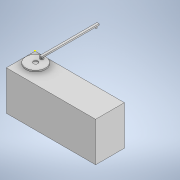
# Autodesk Inventor part: fnal
Saved by Autodesk Inventor 2021 (Build 250183000, 183)
## iProperties
Created: 2021-03-07
Part Number: fnal
Material: Generic
Document SubType Name: Modeling
Designer: V.Basavaraj
Density: 1 g/cm^3
Appearance: Default
Author: V.Basavaraj
Autodesk Inventor part; units mm, degrees
ref_plane "YZ Plane" through (0, 0, 0) normal (1, 0, 0) x (0, 1, 0)
ref_plane "XZ Plane" through (0, 0, 0) normal (0, 1, 0) x (-1, 0, 0)
ref_plane "XY Plane" through (0, 0, 0) normal (0, 0, 1) x (1, 0, 0)
sketch "Sketch1" plane through (0, 0, 0) normal (0, 0, 1) x (1, 0, 0)
  line L0 (0, 0) -> (124.045, 0)
  line L1 (124.045, 0) -> (124.045, -54.7779)
  line L2 (124.045, -54.7779) -> (0, -54.7779)
  line L3 (0, -54.7779) -> (0, 0)
  constraints: 8 end point, 2 parallel, 1 horizontal, 1 perpendicular
extrude "Extrusion1" add sketch "Sketch1" along normal blind 40
sketch "Sketch2" plane through (0, -54.7779, 0) normal (0, -1, 0) x (1, 0, 0)
  circle A0 centre (9.1512, 19.8276) radius 6.8021
  circle A1 centre (8.9796, 19.8276) radius 6.8021
  line L0 (22.4204, 25.1658) -> (80.2254, 25.1658)
  line L1 (80.2254, 25.1658) -> (80.2254, 11.439)
  line L2 (80.2254, 11.439) -> (22.4204, 11.439)
  line L3 (22.4204, 11.439) -> (22.4204, 25.1658)
  line L4 (102.3407, 25.1658) -> (111.1869, 25.1658)
  line L5 (111.1869, 25.1658) -> (111.1869, 11.439)
  line L6 (111.1869, 11.439) -> (102.3407, 11.439)
  line L7 (102.3407, 11.439) -> (102.3407, 25.1658)
  point P0 (0, 0)
  point P1 (9.0654, 26.6291)
  point P2 (9.0654, 13.026)
  constraints: 16 end point, 4 parallel, 2 centre point, 2 horizontal, 2 perpendicular, 2 point on line
extrude "Extrusion2" cut sketch "Sketch2" against normal blind 40 contours A1 A0 | L0 L1 L2 L3 | L4 L5 L6 L7 picked at (6.8592, 19.8276)
sketch "Sketch3" plane through (0, 0, 0) normal (0, 1, 0) x (1, 0, 0)
  circle A0 centre (18.8298, -18.0971) radius 3.199
  arc A1 (9.0654, -26.6291) -> (9.0654, -13.026) centre (8.9796, -19.8276) ccw projected
  point P0 (0, 0)
  constraints: 1 centre point, 1 tangent
extrude "Extrusion3" add sketch "Sketch3" along normal blind 4
sketch "Sketch4" plane through (18.8298, 4, 18.0971) normal (0, 1, 0) x (1, 0, 0)
  circle A0 centre (0, 0) radius 3.199 projected
  circle A1 centre (0, 0) radius 13.6557
  point P0 (-18.8298, 18.0971)
  constraints: 1 centre point, 1 coincident
extrude "Extrusion4" add sketch "Sketch4" along normal mid plane 2
sketch "Sketch5" plane through (18.8298, 5, 18.0971) normal (0, 1, 0) x (1, 0, 0)
  circle A0 centre (-0.2098, 8.868) radius 2.3351
  point P0 (-18.8298, 18.0971)
  constraints: 1 centre point
extrude "Extrusion5" add sketch "Sketch5" along normal blind 2
sketch "Sketch6" plane through (18.62, 7, 9.2291) normal (0, 1, 0) x (1, 0, 0)
  line L0 (1.7734, 77.6649) -> (-1.1678, 77.6649)
  line L1 (-1.1678, 77.6649) -> (-1.1678, -2.3351)
  line L2 (-1.1678, -2.3351) -> (1.7734, -2.3351)
  line L3 (1.7734, -2.3351) -> (1.7734, 77.6649)
  line L4 (1.7734, 77.6649) -> (-1.1678, -2.3351) construction
  line L5 (-1.1678, 77.6649) -> (1.7734, -2.3351) construction
  point P0 (-18.62, 9.2291)
  point P1 (0.3028, 37.6649)
  dimension "d10" = 80
  constraints: 12 end point, 2 midpoint, 2 parallel, 1 horizontal, 1 perpendicular
  measures "d10" distance of L2.end L0.start
extrude "Extrusion6" add sketch "Sketch6" along normal blind 2
sketch "Sketch7" plane through (0, 0, 0) normal (0, 0, -1) x (-1, 0, 0)
  point P0 (0, 0)
sketch "Sketch8" plane through (18.62, 7, 9.2291) normal (0, -1, 0) x (1, 0, 0)
  circle A0 centre (0.5375, -74.8079) radius 1.3827
  point P0 (-18.62, -9.2291)
  constraints: 1 centre point
extrude "Extrusion7" add sketch "Sketch8" along normal blind 2
body "Solid1"
